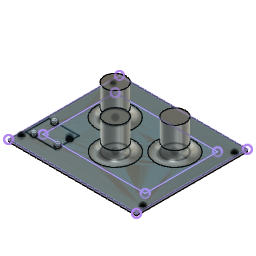
MUS3005bottom (Autodesk Fusion 360 design; units mm, degrees)
Autodesk Fusion 360 part; units mm, degrees
sketch "Sketch1" plane through (0, 0, 0) normal (0, 0, 1) x (1, 0, 0)
  line L0 (0, 0) -> (300, 0)
  line L1 (300, 0) -> (300, 260)
  line L2 (300, 260) -> (0, 260)
  line L3 (0, 260) -> (0, 0)
  dimension "d1" = 300
  dimension "d2" = 260
  constraint horizontal L0
  constraint vertical L1
  constraint horizontal L2
  constraint vertical L3
  constraint coincident L0.start L3.end
  measures "d1" distance of L0.start L0.end
  measures "d2" distance of L0.start L2.end
extrude "Extrude1" add sketch "Sketch1" along normal blind 5
sketch "Sketch2" plane through (0, 0, 5) normal (0, 0, 1) x (-1, 0, 0)
  line L0 (0, -260) -> (0, 0)
  line L1 (0, 0) -> (-300, 0)
  line L2 (-300, 0) -> (-300, -260)
  line L3 (-300, -260) -> (0, -260)
  circle A0 centre (-7.5, -237.5) radius 2.5
  circle A1 centre (-292.5, -237.5) radius 2.5
  circle A2 centre (-7.5, -22.5) radius 2.5
  circle A3 centre (-292.5, -22.5) radius 2.5
  dimension "d5" = 5
  dimension "d6" = 5
  dimension "d7" = 5
  dimension "d8" = 5
  dimension "d9" = 7.5
  dimension "d10" = 22.5
  dimension "d11" = 22.5
  dimension "d12" = 7.5
  dimension "d13" = 22.5
  dimension "d14" = 7.5
  dimension "d15" = 22.5
  dimension "d16" = 7.5
  measures "d5" diameter of A0
  measures "d6" diameter of A1
  measures "d7" diameter of A2
  measures "d8" diameter of A3
  measures "d9" distance of L0 A0.centre
  measures "d10" distance of L3 A0.centre
  measures "d11" distance of L3 A1.centre
  measures "d12" distance of L2 A1.centre
  measures "d13" distance of L1 A3.centre
  measures "d14" distance of L2 A3.centre
  measures "d15" distance of L1 A2.centre
  measures "d16" distance of L0 A2.centre
sketch "Sketch3" plane through (0, 0, 5) normal (0, 0, 1) x (1, 0, 0)
  line L0 (75, 35) -> (5, 35)
  line L1 (5, 35) -> (5, 89.718)
  line L2 (5, 89.718) -> (75, 89.718)
  line L3 (75, 89.718) -> (75, 35)
  line L4 (0, 260) -> (0, 0)
  circle A0 centre (72, 43.118) radius 3
  circle A1 centre (72, 71.018) radius 3
  circle A2 centre (21.2, 38) radius 3
  circle A3 centre (21.2, 86.218) radius 3
  line L5 (0, 0) -> (300, 0)
  line L6 (270, 50.5) -> (30, 50.5)
  line L7 (30, 50.5) -> (30, 220)
  line L8 (30, 220) -> (270, 220)
  line L9 (270, 220) -> (270, 50.5)
  line L10 (300, 260) -> (0, 260)
  line L11 (300, 0) -> (300, 260)
  dimension "d17" = 70
  dimension "d18" = 54.718
  dimension "d19" = 5
  dimension "d20" = 6
  dimension "d21" = 6
  dimension "d22" = 6
  dimension "d23" = 6
  dimension "d24" = 67
  dimension "d25" = 67
  dimension "d26" = 16.2
  dimension "d27" = 16.2
  dimension "d28" = 18.7
  dimension "d29" = 27.9
  dimension "d30" = 3.5
  dimension "d31" = 48.218
  dimension "d32" = 35
  dimension "d33" = 240
  dimension "d34" = 50.5
  dimension "d35" = 169.5
  dimension "d36" = 40
  dimension "d37" = 30
  dimension "d38" = 30
  constraint horizontal L0
  constraint vertical L1
  constraint horizontal L2
  constraint vertical L3
  constraint horizontal L6
  constraint vertical L7
  constraint horizontal L8
  constraint vertical L9
  measures "d17" distance of L0.start L0.end
  measures "d18" distance of L0.start L2.end
  measures "d19" distance of L1 L4
  measures "d20" diameter of A0
  measures "d21" diameter of A1
  measures "d22" diameter of A2
  measures "d23" diameter of A3
  measures "d24" distance of L1 A0.centre
  measures "d25" distance of L1 A1.centre
  measures "d26" distance of L1 A3.centre
  measures "d27" distance of L1 A2.centre
  measures "d28" distance of L2 A1.centre
  measures "d29" distance of A0.centre A1.centre
  measures "d30" distance of L2 A3.centre
  measures "d31" distance of A2.centre A3.centre
  measures "d32" distance of L0 L5
  measures "d33" distance of L6.start L6.end
  measures "d34" distance of L5 L6
  measures "d35" distance of L6.start L8.end
  measures "d36" distance of L8 L10
  measures "d37" distance of L9 L11
  measures "d38" distance of L4 L7
extrude "Extrude2" add sketch "Sketch3" along normal blind 5 contours A0
extrude "Extrude3" add sketch "Sketch3" along normal blind 5 contours A2
extrude "Extrude4" add sketch "Sketch3" along normal blind 5 contours A1
extrude "Extrude5" add sketch "Sketch3" along normal blind 5 contours A3
sketch "Sketch4" plane through (0, 0, 5) normal (0, 0, 1) x (1, 0, 0)
sketch "Sketch5" plane through (0, 0, 10) normal (0, 0, 1) x (-1, 0, 0)
  circle A0 centre (-72, -71.018) radius 3
  circle A1 centre (-72, -71.018) radius 1.5
  circle A2 centre (-71.979, -43.1144) radius 1.5
  circle A3 centre (-21.1713, -38.0167) radius 1.5
  circle A4 centre (-21.1713, -86.1905) radius 1.5
  dimension "d47" = 3
  dimension "d48" = 3
  dimension "d49" = 3
  dimension "d50" = 3
  constraint concentric A0 A1
  measures "d47" diameter of A1
  measures "d48" diameter of A2
  measures "d49" diameter of A3
  measures "d50" diameter of A4
extrude "Extrude6" cut sketch "Sketch5" against normal blind 10 contours A2
extrude "Extrude7" cut sketch "Sketch5" against normal blind 10 contours A1
extrude "Extrude8" cut sketch "Sketch5" against normal blind 10 contours A3
extrude "Extrude9" cut sketch "Sketch5" against normal blind 10 contours A4
extrude "Extrude10" add sketch "Sketch2" along normal blind 20 contours A3
extrude "Extrude11" add sketch "Sketch2" along normal blind 20 contours A1
extrude "Extrude12" add sketch "Sketch2" along normal blind 20 contours A0
extrude "Extrude13" add sketch "Sketch2" along normal blind 20 contours A2
sketch "Sketch6" plane through (0, 0, 5) normal (0, 0, 1) x (1, 0, 0)
  circle A0 centre (80, 170) radius 25
  circle A1 centre (220, 170) radius 25
  circle A2 centre (150, 100.5) radius 25
  line L0 (30, 220) -> (270, 220)
  line L1 (30, 50.5) -> (30, 220)
  line L2 (270, 220) -> (270, 50.5)
  line L3 (270, 50.5) -> (30, 50.5)
  dimension "d67" = 50
  dimension "d68" = 50
  dimension "d69" = 50
  dimension "d70" = 50
  dimension "d71" = 50
  dimension "d72" = 50
  dimension "d73" = 50
  dimension "d74" = 50
  dimension "d75" = 140
  dimension "d76" = 120
  measures "d67" diameter of A0
  measures "d68" diameter of A1
  measures "d69" diameter of A2
  measures "d70" distance of A0.centre L0
  measures "d71" distance of A0.centre L1
  measures "d72" distance of A1.centre L0
  measures "d73" distance of A1.centre L2
  measures "d74" distance of A2.centre L3
  measures "d75" distance of A0.centre A1.centre
  measures "d76" distance of A2.centre L1
extrude "Extrude14" add sketch "Sketch6" along normal blind 75.7 contours A2
extrude "Extrude15" add sketch "Sketch6" along normal blind 75.5 contours A1
extrude "Extrude16" add sketch "Sketch6" along normal blind 75.5 contours A0
sketch "Sketch7" plane through (0, 0, 25) normal (0, 0, 1) x (-1, 0, 0)
  circle A0 centre (-7.5, -237.5) radius 2.5
  circle A1 centre (-7.5, -237.5) radius 2.25
  dimension "d83" = 4.5
  constraint concentric A0 A1
  measures "d83" diameter of A1
sketch "Sketch8" plane through (0, 0, 25) normal (0, 0, 1) x (-1, 0, 0)
  circle A0 centre (-292.5, -237.5) radius 2.5
  circle A1 centre (-292.5, -237.5) radius 2.25
  dimension "d84" = 4.5
  constraint concentric A0 A1
  measures "d84" diameter of A1
extrude "Extrude17" cut sketch "Sketch8" against normal blind 20
extrude "Extrude18" cut sketch "Sketch7" against normal blind 20
sketch "Sketch9" plane through (0, 0, 25) normal (0, 0, 1) x (-1, 0, 0)
  circle A0 centre (-7.5, -22.5) radius 2.5
  circle A1 centre (-7.5, -22.5) radius 2.25
  dimension "d89" = 4.5
  constraint concentric A0 A1
  measures "d89" diameter of A1
extrude "Extrude19" cut sketch "Sketch9" against normal blind 20
sketch "Sketch10" plane through (0, 0, 25) normal (0, 0, 1) x (-1, 0, 0)
  circle A0 centre (-292.5, -22.5) radius 2.5
  circle A1 centre (-292.5, -22.5) radius 2.25
  dimension "d92" = 4.5
  constraint concentric A0 A1
  measures "d92" diameter of A1
extrude "Extrude20" cut sketch "Sketch10" against normal blind 20
fillet "Fillet1" radius 2.5 4 edges at (18.403, 39.0848, 5) (69.203, 44.2028, 5) (69.203, 72.1028, 5) (18.403, 87.3028, 5)
fillet "Fillet2" radius 20 3 edges at (126.6918, 109.5404, 5) (56.6918, 179.0404, 5) (196.6918, 179.0404, 5)
extrude "Extrude21" cut 1 faces at (221.8543, 161.8756, 80.5) along direction (0, 0, -1) blind 4
extrude "Extrude22" cut 1 faces at (146.1592, 99.9211, 80.7) along direction (0, 0, -1) blind 4
extrude "Extrude23" cut 1 faces at (85.1957, 176.5153, 80.5) along direction (0, 0, -1) blind 4
extrude "Extrude24" cut 1 faces at (7.0129, 238.1495, 25) along direction (0, 0, -1) blind 25
extrude "Extrude25" cut 1 faces at (8.0831, 23.2312, 25) along direction (0, 0, -1) blind 25
extrude "Extrude26" cut 1 faces at (291.0333, 22.7211, 25) along direction (0, 0, -1) blind 25
extrude "Extrude27" cut 1 faces at (294.0593, 237.2158, 25) along direction (0, 0, -1) blind 25
